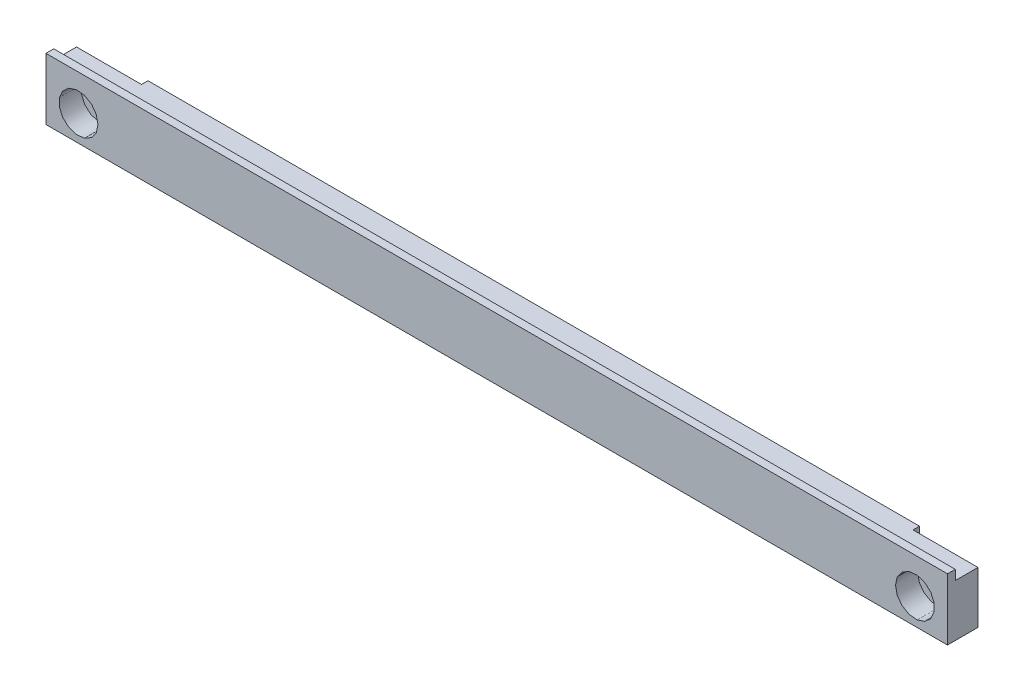
# Autodesk Inventor part: Case_bottom_front
Saved by Autodesk Inventor 2016 SP2 (Build 200236200, 236)
## iProperties
Created: 2018-06-26
Part Number: Case_bottom_front
Material: Generisch
Document SubType Name: Modeling
Designer: Nils
Density: 1 g/cm^3
Appearance: Vorgabe
Author: Nils
Autodesk Inventor part; units mm, degrees
ref_plane "YZ Plane" through (0, 0, 0) normal (1, 0, 0) x (0, 1, 0)
ref_plane "XZ Plane" through (0, 0, 0) normal (0, 1, 0) x (-1, 0, 0)
ref_plane "XY Plane" through (0, 0, 0) normal (0, 0, 1) x (1, 0, 0)
sketch "Skizze2" plane through (0, 0, 0) normal (1, 0, 0) x (0, 1, 0)
  line L0 (33.2284, 10.7468) -> (33.2284, 9.7468)
  line L1 (33.2284, 10.7468) -> (33.2284, 15.4468)
  line L2 (33.2284, 15.4468) -> (42.7284, 15.4468)
  line L3 (41.2284, 9.7468) -> (33.2284, 9.7468)
  line L4 (42.7284, 14.2468) -> (41.2284, 14.2468)
  line L5 (42.7284, 14.2468) -> (42.7284, 15.4468)
  line L6 (33.2284, 15.4468) -> (42.7284, 15.4468)
  line L7 (33.2284, 10.7468) -> (33.2284, 15.4468)
  line L8 (33.2284, 10.7468) -> (41.2284, 10.7468)
  line L9 (41.2284, 14.2468) -> (41.2284, 10.7468)
  line L10 (42.7284, 14.2468) -> (42.7284, 15.4468)
  line L11 (41.2284, 10.7468) -> (41.2284, 9.7468)
  point P0 (0, 0)
extrude "Extrusion1" add sketch "Skizze2" along normal blind 69.4
sketch "Skizze3" plane through (0, 0, 0) normal (-1, 0, 0) x (0, 0, 1)
  line L0 (14.2468, 42.7284) -> (14.2468, 41.2284) projected
  line L1 (14.2468, 42.7284) -> (15.4468, 42.7284) projected
  line L2 (15.4468, 33.2284) -> (15.4468, 42.7284) projected
  line L3 (10.7468, 33.2284) -> (15.4468, 33.2284) projected
  line L4 (10.7468, 33.2284) -> (10.7468, 41.2284) projected
  line L5 (14.2468, 41.2284) -> (10.7468, 41.2284) projected
  line L6 (9.7468, 33.2284) -> (9.7468, 41.2284) projected
  line L7 (9.7468, 41.2284) -> (10.7468, 41.2284)
  line L8 (10.7468, 41.2284) -> (10.7468, 33.2284)
  line L9 (10.7468, 33.2284) -> (9.7468, 33.2284)
  line L10 (9.7468, 33.2284) -> (9.7468, 41.2284)
  point P0 (0, 0)
  constraints: 8 end point, 2 parallel, 1 horizontal, 1 perpendicular
extrude "Extrusion2" cut sketch "Skizze3" against normal blind 10 contours L4 L9 L6 L7
sketch "Skizze4" plane through (0, 33.2284, 15.4468) normal (0, 0, 1) x (1, 0, 0)
  line L0 (0, 0) -> (10, 0) construction
  line L1 (5, 0) -> (5, 9.5) construction
  line L2 (0, 9.5) -> (69.4, 9.5) construction
  circle A0 centre (5, 4) radius 3
  line L3 (0, 9.5) -> (0, 0) construction
  point P0 (0, -33.2284)
  dimension "d4" = 6
  dimension "d5" = 5
  dimension "d6" = 4
  constraints: 2 end point, 2 point on line, 1 centre point, 1 midpoint, 1 vertical
  measures "d4" diameter of A0
  measures "d5" distance between parallel lines of L3 L1
  measures "d6" distance from line of L0 A0.centre
extrude "Extrusion3" cut sketch "Skizze4" against normal blind 3.4
sketch "Skizze5" plane through (5, 37.2284, 12.0468) normal (0, 0, 1) x (1, 0, 0)
  circle A0 centre (0, 0) radius 3 projected
  circle A1 centre (0, 0) radius 1.75
  point P0 (-5, -37.2284)
  dimension "d9" = 3.5
  constraints: 1 centre point, 1 coincident
  measures "d9" diameter of A1
extrude "Extrusion4" cut sketch "Skizze5" against normal blind 3.4 contours A1
mirror "Spiegeln1" about plane through (69.4, 37.2284, 10.2468) normal (1, 0, 0) of "Extrusion4", "Extrusion3", "Extrusion2", "Extrusion1"
